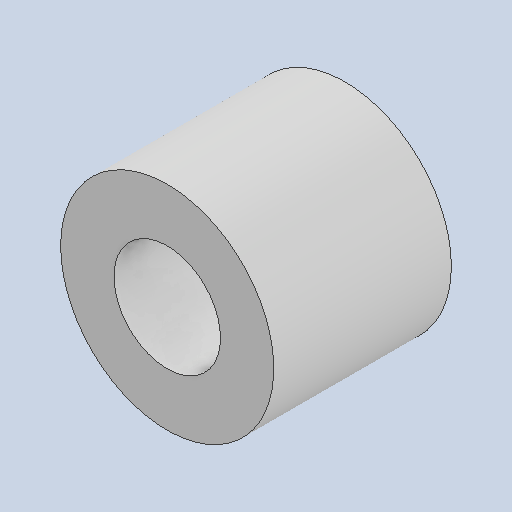
# Autodesk Inventor part: plate_3_washers
Saved by Autodesk Inventor 2024 (Build 280153000, 153)
## iProperties
Created: 2026-02-08
Part Number: plate_3_washers
Material: Generic
Document SubType Name: Modeling
Designer: SEMEN
Density: 1 g/cm^3
Appearance: Default
Author: SEMEN
Autodesk Inventor part; units mm, degrees
ref_plane "YZ Plane" through (0, 0, 0) normal (1, 0, 0) x (0, 1, 0)
ref_plane "XZ Plane" through (0, 0, 0) normal (0, 1, 0) x (-1, 0, 0)
ref_plane "Work Plane1" through (-100.1793, -14.2479, 10) normal (0, 0, -1) x (0, 1, 0)
sketch "Sketch1" plane through (0, 0, 0) normal (0, 0, 1) x (1, 0, 0)
  circle A0 centre (-90.1793, 21.1555) radius 2.5 projected
  circle A1 centre (-90.1793, 21.1555) radius 10 projected
  circle A2 centre (-90.1793, 21.1555) radius 3
  circle A3 centre (-90.1793, 21.1555) radius 6
  point P0 (0, 0)
  dimension "d0" = 0.5
  dimension "d1" = 3
  constraints: 2 centre point
  measures "d0" radial gap between concentric circles of A0 A2
  measures "d1" radial gap between concentric circles of A2 A3
extrude "Extrusion1" add sketch "Sketch1" along normal up to surface (10 mm away) contours A3
body "Solid1"
